Autodesk Fusion 360 part; units mm, degrees
note: some values were not read from the file. Set by a fixed rule: which sketch regions a step uses.
(part 2 of 3)
sketch "Schizzo100" plane through (0, 18, -31.1769) normal (0, 0.5, -0.866025) x (0, -0.866025, -0.5)
  circle A0 centre (14.956, -5.5311) radius 0.5023
  circle A1 centre (14.956, -9.1821) radius 0.5023
  circle A2 centre (14.956, -12.833) radius 0.5023
  circle A3 centre (14.956, -16.4839) radius 0.5023
  circle A4 centre (14.956, -20.1349) radius 0.5023
  circle A5 centre (14.956, -23.7858) radius 0.5023
  circle A6 centre (14.956, -27.4367) radius 0.5023
  circle A7 centre (14.956, -31.0877) radius 0.5023
  circle A8 centre (14.956, -34.7386) radius 0.5023
  circle A9 centre (14.956, -38.3895) radius 0.5023
  circle A10 centre (14.956, -42.0405) radius 0.5023
  circle A11 centre (14.956, -45.6914) radius 0.5023
  circle A12 centre (14.956, -49.3423) radius 0.5023
  circle A13 centre (14.956, -52.9933) radius 0.5023
  circle A14 centre (14.956, -56.6442) radius 0.5023
  circle A15 centre (14.956, -60.2951) radius 0.5023
  circle A16 centre (14.956, -63.9461) radius 0.5023
  circle A17 centre (14.956, -67.597) radius 0.5023
  circle A18 centre (14.956, -71.248) radius 0.5023
  circle A19 centre (14.956, -74.8989) radius 0.5023
  circle A20 centre (14.956, -78.5498) radius 0.5023
  circle A21 centre (14.956, -82.2008) radius 0.5023
  circle A22 centre (14.956, -85.8517) radius 0.5023
  circle A23 centre (14.956, -89.5026) radius 0.5023
  circle A24 centre (14.956, -93.1536) radius 0.5023
  circle A25 centre (14.956, -96.8045) radius 0.5023
  circle A26 centre (14.956, -100.4554) radius 0.5023
  circle A27 centre (14.956, -104.1064) radius 0.5023
  circle A28 centre (14.956, -107.7573) radius 0.5023
  circle A29 centre (14.956, -111.4082) radius 0.5023
  circle A30 centre (14.956, -115.0592) radius 0.5023
  circle A31 centre (14.956, -118.7101) radius 0.5023
  circle A32 centre (14.956, -122.361) radius 0.5023
  circle A33 centre (14.956, -126.012) radius 0.5023
  circle A34 centre (14.956, -129.6629) radius 0.5023
  circle A35 centre (14.956, -133.3138) radius 0.5023
  circle A36 centre (14.956, -136.9648) radius 0.5023
  circle A37 centre (14.956, -140.6157) radius 0.5023
  circle A38 centre (14.956, -144.2667) radius 0.5023
  circle A39 centre (14.956, -147.9176) radius 0.5023
  circle A40 centre (14.956, -151.5685) radius 0.5023
  circle A41 centre (14.956, -155.2195) radius 0.5023
  circle A42 centre (14.956, -158.8704) radius 0.5023
  circle A43 centre (14.956, -162.5213) radius 0.5023
  circle A44 centre (14.956, -166.1723) radius 0.5023
  circle A45 centre (14.956, -169.8232) radius 0.5023
  circle A46 centre (14.956, -173.4741) radius 0.5023
  circle A47 centre (14.956, -177.1251) radius 0.5023
  circle A48 centre (14.956, -180.776) radius 0.5023
  circle A49 centre (14.956, -184.4269) radius 0.5023
  circle A50 centre (14.956, -188.0779) radius 0.5023
  circle A51 centre (14.956, -191.7288) radius 0.5023
  circle A52 centre (14.956, -195.3797) radius 0.5023
  circle A53 centre (14.956, -199.0307) radius 0.5023
  circle A54 centre (14.956, -202.6816) radius 0.5023
  circle A55 centre (14.956, -206.3325) radius 0.5023
  circle A56 centre (14.956, -209.9835) radius 0.5023
  circle A57 centre (14.956, -213.6344) radius 0.5023
  circle A58 centre (14.956, -217.2853) radius 0.5023
  circle A59 centre (14.956, -220.9363) radius 0.5023
  circle A60 centre (14.956, -224.5872) radius 0.5023
  circle A61 centre (13.1468, -7.3404) radius 0.5023
  circle A62 centre (13.1468, -10.9913) radius 0.5023
  circle A63 centre (13.1468, -14.6422) radius 0.5023
  circle A64 centre (13.1468, -18.2932) radius 0.5023
  circle A65 centre (13.1468, -21.9441) radius 0.5023
  circle A66 centre (13.1468, -25.595) radius 0.5023
  circle A67 centre (13.1468, -29.246) radius 0.5023
  circle A68 centre (13.1468, -32.8969) radius 0.5023
  circle A69 centre (13.1468, -36.5478) radius 0.5023
  circle A70 centre (13.1468, -40.1988) radius 0.5023
  circle A71 centre (13.1468, -43.8497) radius 0.5023
  circle A72 centre (13.1468, -47.5006) radius 0.5023
  circle A73 centre (13.1468, -51.1516) radius 0.5023
  circle A74 centre (13.1468, -54.8025) radius 0.5023
  circle A75 centre (13.1468, -58.4534) radius 0.5023
  circle A76 centre (13.1468, -62.1044) radius 0.5023
  circle A77 centre (13.1468, -65.7553) radius 0.5023
  circle A78 centre (13.1468, -69.4062) radius 0.5023
  circle A79 centre (13.1468, -73.0572) radius 0.5023
  circle A80 centre (13.1468, -76.7081) radius 0.5023
  circle A81 centre (13.1468, -80.3591) radius 0.5023
  circle A82 centre (13.1468, -84.01) radius 0.5023
  circle A83 centre (13.1468, -87.6609) radius 0.5023
  circle A84 centre (13.1468, -91.3119) radius 0.5023
  circle A85 centre (13.1468, -94.9628) radius 0.5023
  circle A86 centre (13.1468, -98.6137) radius 0.5023
  circle A87 centre (13.1468, -102.2647) radius 0.5023
  circle A88 centre (13.1468, -105.9156) radius 0.5023
  circle A89 centre (13.1468, -109.5665) radius 0.5023
  circle A90 centre (13.1468, -113.2175) radius 0.5023
  circle A91 centre (13.1468, -116.8684) radius 0.5023
  circle A92 centre (13.1468, -120.5193) radius 0.5023
  circle A93 centre (13.1468, -124.1703) radius 0.5023
  circle A94 centre (13.1468, -127.8212) radius 0.5023
  circle A95 centre (13.1468, -131.4721) radius 0.5023
  circle A96 centre (13.1468, -135.1231) radius 0.5023
  circle A97 centre (13.1468, -138.774) radius 0.5023
  circle A98 centre (13.1468, -142.4249) radius 0.5023
  circle A99 centre (13.1468, -146.0759) radius 0.5023
  circle A100 centre (13.1468, -149.7268) radius 0.5023
  circle A101 centre (13.1468, -153.3778) radius 0.5023
  circle A102 centre (13.1468, -157.0287) radius 0.5023
  circle A103 centre (13.1468, -160.6796) radius 0.5023
  circle A104 centre (13.1468, -164.3306) radius 0.5023
  circle A105 centre (13.1468, -167.9815) radius 0.5023
  circle A106 centre (13.1468, -171.6324) radius 0.5023
  circle A107 centre (13.1468, -175.2834) radius 0.5023
  circle A108 centre (13.1468, -178.9343) radius 0.5023
  circle A109 centre (13.1468, -182.5852) radius 0.5023
  circle A110 centre (13.1468, -186.2362) radius 0.5023
  circle A111 centre (13.1468, -189.8871) radius 0.5023
  circle A112 centre (13.1468, -193.538) radius 0.5023
  circle A113 centre (13.1468, -197.189) radius 0.5023
  circle A114 centre (13.1468, -200.8399) radius 0.5023
  circle A115 centre (13.1468, -204.4908) radius 0.5023
  circle A116 centre (13.1468, -208.1418) radius 0.5023
  circle A117 centre (13.1468, -211.7927) radius 0.5023
  circle A118 centre (13.1468, -215.4436) radius 0.5023
  circle A119 centre (13.1468, -219.0946) radius 0.5023
  circle A120 centre (13.1468, -222.7455) radius 0.5023
  circle A121 centre (10.6739, -5.5311) radius 0.5023
  circle A122 centre (10.6739, -9.1821) radius 0.5023
  circle A123 centre (10.6739, -12.833) radius 0.5023
  circle A124 centre (10.6739, -16.4839) radius 0.5023
  circle A125 centre (10.6739, -20.1349) radius 0.5023
  circle A126 centre (10.6739, -23.7858) radius 0.5023
  circle A127 centre (10.6739, -27.4367) radius 0.5023
  circle A128 centre (10.6739, -31.0877) radius 0.5023
  circle A129 centre (10.6739, -34.7386) radius 0.5023
  circle A130 centre (10.6739, -38.3895) radius 0.5023
  circle A131 centre (10.6739, -42.0405) radius 0.5023
  circle A132 centre (10.6739, -45.6914) radius 0.5023
  circle A133 centre (10.6739, -49.3423) radius 0.5023
  circle A134 centre (10.6739, -52.9933) radius 0.5023
  circle A135 centre (10.6739, -56.6442) radius 0.5023
  circle A136 centre (10.6739, -60.2951) radius 0.5023
  circle A137 centre (10.6739, -63.9461) radius 0.5023
  circle A138 centre (10.6739, -67.597) radius 0.5023
  circle A139 centre (10.6739, -71.248) radius 0.5023
  circle A140 centre (10.6739, -74.8989) radius 0.5023
  circle A141 centre (10.6739, -78.5498) radius 0.5023
  circle A142 centre (10.6739, -82.2008) radius 0.5023
  circle A143 centre (10.6739, -85.8517) radius 0.5023
  circle A144 centre (10.6739, -89.5026) radius 0.5023
  circle A145 centre (10.6739, -93.1536) radius 0.5023
  circle A146 centre (10.6739, -96.8045) radius 0.5023
  circle A147 centre (10.6739, -100.4554) radius 0.5023
  circle A148 centre (10.6739, -104.1064) radius 0.5023
  circle A149 centre (10.6739, -107.7573) radius 0.5023
  circle A150 centre (10.6739, -111.4082) radius 0.5023
  circle A151 centre (10.6739, -115.0592) radius 0.5023
  circle A152 centre (10.6739, -118.7101) radius 0.5023
  circle A153 centre (10.6739, -122.361) radius 0.5023
  circle A154 centre (10.6739, -126.012) radius 0.5023
  circle A155 centre (10.6739, -129.6629) radius 0.5023
  circle A156 centre (10.6739, -133.3138) radius 0.5023
  circle A157 centre (10.6739, -136.9648) radius 0.5023
  circle A158 centre (10.6739, -140.6157) radius 0.5023
  circle A159 centre (10.6739, -144.2667) radius 0.5023
  circle A160 centre (10.6739, -147.9176) radius 0.5023
  circle A161 centre (10.6739, -151.5685) radius 0.5023
  circle A162 centre (10.6739, -155.2195) radius 0.5023
  circle A163 centre (10.6739, -158.8704) radius 0.5023
  circle A164 centre (10.6739, -162.5213) radius 0.5023
  circle A165 centre (10.6739, -166.1723) radius 0.5023
  circle A166 centre (10.6739, -169.8232) radius 0.5023
  circle A167 centre (10.6739, -173.4741) radius 0.5023
  circle A168 centre (10.6739, -177.1251) radius 0.5023
  circle A169 centre (10.6739, -180.776) radius 0.5023
  circle A170 centre (10.6739, -184.4269) radius 0.5023
  circle A171 centre (10.6739, -188.0779) radius 0.5023
  circle A172 centre (10.6739, -191.7288) radius 0.5023
  circle A173 centre (10.6739, -195.3797) radius 0.5023
  circle A174 centre (10.6739, -199.0307) radius 0.5023
  circle A175 centre (10.6739, -202.6816) radius 0.5023
  circle A176 centre (10.6739, -206.3325) radius 0.5023
  circle A177 centre (10.6739, -209.9835) radius 0.5023
  circle A178 centre (10.6739, -213.6344) radius 0.5023
  circle A179 centre (10.6739, -217.2853) radius 0.5023
  circle A180 centre (10.6739, -220.9363) radius 0.5023
  circle A181 centre (10.6739, -224.5872) radius 0.5023
  circle A182 centre (8.8647, -7.3404) radius 0.5023
  circle A183 centre (8.8647, -10.9913) radius 0.5023
  circle A184 centre (8.8647, -14.6422) radius 0.5023
  circle A185 centre (8.8647, -18.2932) radius 0.5023
  circle A186 centre (8.8647, -21.9441) radius 0.5023
  circle A187 centre (8.8647, -25.595) radius 0.5023
  circle A188 centre (8.8647, -29.246) radius 0.5023
  circle A189 centre (8.8647, -32.8969) radius 0.5023
  circle A190 centre (8.8647, -36.5478) radius 0.5023
  circle A191 centre (8.8647, -40.1988) radius 0.5023
  circle A192 centre (8.8647, -43.8497) radius 0.5023
  circle A193 centre (8.8647, -47.5006) radius 0.5023
  circle A194 centre (8.8647, -51.1516) radius 0.5023
  circle A195 centre (8.8647, -54.8025) radius 0.5023
  circle A196 centre (8.8647, -58.4534) radius 0.5023
  circle A197 centre (8.8647, -62.1044) radius 0.5023
  circle A198 centre (8.8647, -65.7553) radius 0.5023
  circle A199 centre (8.8647, -69.4062) radius 0.5023
  circle A200 centre (8.8647, -73.0572) radius 0.5023
  circle A201 centre (8.8647, -76.7081) radius 0.5023
  circle A202 centre (8.8647, -80.3591) radius 0.5023
  circle A203 centre (8.8647, -84.01) radius 0.5023
  circle A204 centre (8.8647, -87.6609) radius 0.5023
  circle A205 centre (8.8647, -91.3119) radius 0.5023
  circle A206 centre (8.8647, -94.9628) radius 0.5023
  circle A207 centre (8.8647, -98.6137) radius 0.5023
  circle A208 centre (8.8647, -102.2647) radius 0.5023
  circle A209 centre (8.8647, -105.9156) radius 0.5023
  circle A210 centre (8.8647, -109.5665) radius 0.5023
  circle A211 centre (8.8647, -113.2175) radius 0.5023
  circle A212 centre (8.8647, -116.8684) radius 0.5023
  circle A213 centre (8.8647, -120.5193) radius 0.5023
  circle A214 centre (8.8647, -124.1703) radius 0.5023
  circle A215 centre (8.8647, -127.8212) radius 0.5023
  circle A216 centre (8.8647, -131.4721) radius 0.5023
  circle A217 centre (8.8647, -135.1231) radius 0.5023
  circle A218 centre (8.8647, -138.774) radius 0.5023
  circle A219 centre (8.8647, -142.4249) radius 0.5023
  circle A220 centre (8.8647, -146.0759) radius 0.5023
  circle A221 centre (8.8647, -149.7268) radius 0.5023
  circle A222 centre (8.8647, -153.3778) radius 0.5023
  circle A223 centre (8.8647, -157.0287) radius 0.5023
  circle A224 centre (8.8647, -160.6796) radius 0.5023
  circle A225 centre (8.8647, -164.3306) radius 0.5023
  circle A226 centre (8.8647, -167.9815) radius 0.5023
  circle A227 centre (8.8647, -171.6324) radius 0.5023
  circle A228 centre (8.8647, -175.2834) radius 0.5023
  circle A229 centre (8.8647, -178.9343) radius 0.5023
  circle A230 centre (8.8647, -182.5852) radius 0.5023
  circle A231 centre (8.8647, -186.2362) radius 0.5023
  circle A232 centre (8.8647, -189.8871) radius 0.5023
  circle A233 centre (8.8647, -193.538) radius 0.5023
  circle A234 centre (8.8647, -197.189) radius 0.5023
  circle A235 centre (8.8647, -200.8399) radius 0.5023
  circle A236 centre (8.8647, -204.4908) radius 0.5023
  circle A237 centre (8.8647, -208.1418) radius 0.5023
  circle A238 centre (8.8647, -211.7927) radius 0.5023
  circle A239 centre (8.8647, -215.4436) radius 0.5023
  circle A240 centre (8.8647, -219.0946) radius 0.5023
  circle A241 centre (8.8647, -222.7455) radius 0.5023
  circle A242 centre (6.3918, -5.5311) radius 0.5023
  circle A243 centre (6.3918, -9.1821) radius 0.5023
  circle A244 centre (6.3918, -12.833) radius 0.5023
  circle A245 centre (6.3918, -16.4839) radius 0.5023
  circle A246 centre (6.3918, -20.1349) radius 0.5023
  circle A247 centre (6.3918, -23.7858) radius 0.5023
  circle A248 centre (6.3918, -27.4367) radius 0.5023
  circle A249 centre (6.3918, -31.0877) radius 0.5023
  circle A250 centre (6.3918, -34.7386) radius 0.5023
  circle A251 centre (6.3918, -38.3895) radius 0.5023
  circle A252 centre (6.3918, -42.0405) radius 0.5023
  circle A253 centre (6.3918, -45.6914) radius 0.5023
  circle A254 centre (6.3918, -49.3423) radius 0.5023
  circle A255 centre (6.3918, -52.9933) radius 0.5023
  circle A256 centre (6.3918, -56.6442) radius 0.5023
  circle A257 centre (6.3918, -60.2951) radius 0.5023
  circle A258 centre (6.3918, -63.9461) radius 0.5023
  circle A259 centre (6.3918, -67.597) radius 0.5023
  circle A260 centre (6.3918, -71.248) radius 0.5023
  circle A261 centre (6.3918, -74.8989) radius 0.5023
  circle A262 centre (6.3918, -78.5498) radius 0.5023
  circle A263 centre (6.3918, -82.2008) radius 0.5023
  circle A264 centre (6.3918, -85.8517) radius 0.5023
  circle A265 centre (6.3918, -89.5026) radius 0.5023
  circle A266 centre (6.3918, -93.1536) radius 0.5023
  circle A267 centre (6.3918, -96.8045) radius 0.5023
  circle A268 centre (6.3918, -100.4554) radius 0.5023
  circle A269 centre (6.3918, -104.1064) radius 0.5023
  circle A270 centre (6.3918, -107.7573) radius 0.5023
  circle A271 centre (6.3918, -111.4082) radius 0.5023
  circle A272 centre (6.3918, -115.0592) radius 0.5023
  circle A273 centre (6.3918, -118.7101) radius 0.5023
  circle A274 centre (6.3918, -122.361) radius 0.5023
  circle A275 centre (6.3918, -126.012) radius 0.5023
  circle A276 centre (6.3918, -129.6629) radius 0.5023
  circle A277 centre (6.3918, -133.3138) radius 0.5023
  circle A278 centre (6.3918, -136.9648) radius 0.5023
  circle A279 centre (6.3918, -140.6157) radius 0.5023
  circle A280 centre (6.3918, -144.2667) radius 0.5023
  circle A281 centre (6.3918, -147.9176) radius 0.5023
  circle A282 centre (6.3918, -151.5685) radius 0.5023
  circle A283 centre (6.3918, -155.2195) radius 0.5023
  circle A284 centre (6.3918, -158.8704) radius 0.5023
  circle A285 centre (6.3918, -162.5213) radius 0.5023
  circle A286 centre (6.3918, -166.1723) radius 0.5023
  circle A287 centre (6.3918, -169.8232) radius 0.5023
  circle A288 centre (6.3918, -173.4741) radius 0.5023
  circle A289 centre (6.3918, -177.1251) radius 0.5023
  circle A290 centre (6.3918, -180.776) radius 0.5023
  circle A291 centre (6.3918, -184.4269) radius 0.5023
  circle A292 centre (6.3918, -188.0779) radius 0.5023
  circle A293 centre (6.3918, -191.7288) radius 0.5023
  circle A294 centre (6.3918, -195.3797) radius 0.5023
  circle A295 centre (6.3918, -199.0307) radius 0.5023
  circle A296 centre (6.3918, -202.6816) radius 0.5023
  circle A297 centre (6.3918, -206.3325) radius 0.5023
  circle A298 centre (6.3918, -209.9835) radius 0.5023
  circle A299 centre (6.3918, -213.6344) radius 0.5023
  circle A300 centre (6.3918, -217.2853) radius 0.5023
  circle A301 centre (6.3918, -220.9363) radius 0.5023
  circle A302 centre (6.3918, -224.5872) radius 0.5023
  circle A303 centre (4.5826, -7.3404) radius 0.5023
  circle A304 centre (4.5826, -10.9913) radius 0.5023
  circle A305 centre (4.5826, -14.6422) radius 0.5023
  circle A306 centre (4.5826, -18.2932) radius 0.5023
  circle A307 centre (4.5826, -21.9441) radius 0.5023
  circle A308 centre (4.5826, -25.595) radius 0.5023
  circle A309 centre (4.5826, -29.246) radius 0.5023
  circle A310 centre (4.5826, -32.8969) radius 0.5023
  circle A311 centre (4.5826, -36.5478) radius 0.5023
  circle A312 centre (4.5826, -40.1988) radius 0.5023
  circle A313 centre (4.5826, -43.8497) radius 0.5023
  circle A314 centre (4.5826, -47.5006) radius 0.5023
  circle A315 centre (4.5826, -51.1516) radius 0.5023
  circle A316 centre (4.5826, -54.8025) radius 0.5023
  circle A317 centre (4.5826, -58.4534) radius 0.5023
  circle A318 centre (4.5826, -62.1044) radius 0.5023
  circle A319 centre (4.5826, -65.7553) radius 0.5023
  circle A320 centre (4.5826, -69.4062) radius 0.5023
  circle A321 centre (4.5826, -73.0572) radius 0.5023
  circle A322 centre (4.5826, -76.7081) radius 0.5023
  circle A323 centre (4.5826, -80.3591) radius 0.5023
  circle A324 centre (4.5826, -84.01) radius 0.5023
  circle A325 centre (4.5826, -87.6609) radius 0.5023
  circle A326 centre (4.5826, -91.3119) radius 0.5023
  circle A327 centre (4.5826, -94.9628) radius 0.5023
  circle A328 centre (4.5826, -98.6137) radius 0.5023
  circle A329 centre (4.5826, -102.2647) radius 0.5023
  circle A330 centre (4.5826, -105.9156) radius 0.5023
  circle A331 centre (4.5826, -109.5665) radius 0.5023
  circle A332 centre (4.5826, -113.2175) radius 0.5023
  circle A333 centre (4.5826, -116.8684) radius 0.5023
  circle A334 centre (4.5826, -120.5193) radius 0.5023
  circle A335 centre (4.5826, -124.1703) radius 0.5023
  circle A336 centre (4.5826, -127.8212) radius 0.5023
  circle A337 centre (4.5826, -131.4721) radius 0.5023
  circle A338 centre (4.5826, -135.1231) radius 0.5023
  circle A339 centre (4.5826, -138.774) radius 0.5023
  circle A340 centre (4.5826, -142.4249) radius 0.5023
  circle A341 centre (4.5826, -146.0759) radius 0.5023
  circle A342 centre (4.5826, -149.7268) radius 0.5023
  circle A343 centre (4.5826, -153.3778) radius 0.5023
  circle A344 centre (4.5826, -157.0287) radius 0.5023
  circle A345 centre (4.5826, -160.6796) radius 0.5023
  circle A346 centre (4.5826, -164.3306) radius 0.5023
  circle A347 centre (4.5826, -167.9815) radius 0.5023
  circle A348 centre (4.5826, -171.6324) radius 0.5023
  circle A349 centre (4.5826, -175.2834) radius 0.5023
  circle A350 centre (4.5826, -178.9343) radius 0.5023
  circle A351 centre (4.5826, -182.5852) radius 0.5023
  circle A352 centre (4.5826, -186.2362) radius 0.5023
  circle A353 centre (4.5826, -189.8871) radius 0.5023
  circle A354 centre (4.5826, -193.538) radius 0.5023
  circle A355 centre (4.5826, -197.189) radius 0.5023
  circle A356 centre (4.5826, -200.8399) radius 0.5023
  circle A357 centre (4.5826, -204.4908) radius 0.5023
  circle A358 centre (4.5826, -208.1418) radius 0.5023
  circle A359 centre (4.5826, -211.7927) radius 0.5023
  circle A360 centre (4.5826, -215.4436) radius 0.5023
  circle A361 centre (4.5826, -219.0946) radius 0.5023
  circle A362 centre (4.5826, -222.7455) radius 0.5023
  circle A363 centre (2.1097, -5.5311) radius 0.5023
  circle A364 centre (2.1097, -9.1821) radius 0.5023
  circle A365 centre (2.1097, -12.833) radius 0.5023
  circle A366 centre (2.1097, -16.4839) radius 0.5023
  circle A367 centre (2.1097, -20.1349) radius 0.5023
  circle A368 centre (2.1097, -23.7858) radius 0.5023
  circle A369 centre (2.1097, -27.4367) radius 0.5023
  circle A370 centre (2.1097, -31.0877) radius 0.5023
  circle A371 centre (2.1097, -34.7386) radius 0.5023
  circle A372 centre (2.1097, -38.3895) radius 0.5023
  circle A373 centre (2.1097, -42.0405) radius 0.5023
  circle A374 centre (2.1097, -45.6914) radius 0.5023
  circle A375 centre (2.1097, -49.3423) radius 0.5023
  circle A376 centre (2.1097, -52.9933) radius 0.5023
  circle A377 centre (2.1097, -56.6442) radius 0.5023
  circle A378 centre (2.1097, -60.2951) radius 0.5023
  circle A379 centre (2.1097, -63.9461) radius 0.5023
  circle A380 centre (2.1097, -67.597) radius 0.5023
  circle A381 centre (2.1097, -71.248) radius 0.5023
  circle A382 centre (2.1097, -74.8989) radius 0.5023
  circle A383 centre (2.1097, -78.5498) radius 0.5023
  circle A384 centre (2.1097, -82.2008) radius 0.5023
  circle A385 centre (2.1097, -85.8517) radius 0.5023
  circle A386 centre (2.1097, -89.5026) radius 0.5023
  circle A387 centre (2.1097, -93.1536) radius 0.5023
  circle A388 centre (2.1097, -96.8045) radius 0.5023
  circle A389 centre (2.1097, -100.4554) radius 0.5023
  circle A390 centre (2.1097, -104.1064) radius 0.5023
  circle A391 centre (2.1097, -107.7573) radius 0.5023
  circle A392 centre (2.1097, -111.4082) radius 0.5023
  circle A393 centre (2.1097, -115.0592) radius 0.5023
  circle A394 centre (2.1097, -118.7101) radius 0.5023
  circle A395 centre (2.1097, -122.361) radius 0.5023
  circle A396 centre (2.1097, -126.012) radius 0.5023
  circle A397 centre (2.1097, -129.6629) radius 0.5023
  circle A398 centre (2.1097, -133.3138) radius 0.5023
  circle A399 centre (2.1097, -136.9648) radius 0.5023
  circle A400 centre (2.1097, -140.6157) radius 0.5023
  circle A401 centre (2.1097, -144.2667) radius 0.5023
  circle A402 centre (2.1097, -147.9176) radius 0.5023
  circle A403 centre (2.1097, -151.5685) radius 0.5023
  circle A404 centre (2.1097, -155.2195) radius 0.5023
  circle A405 centre (2.1097, -158.8704) radius 0.5023
  circle A406 centre (2.1097, -162.5213) radius 0.5023
  circle A407 centre (2.1097, -166.1723) radius 0.5023
  circle A408 centre (2.1097, -169.8232) radius 0.5023
  circle A409 centre (2.1097, -173.4741) radius 0.5023
  circle A410 centre (2.1097, -177.1251) radius 0.5023
  circle A411 centre (2.1097, -180.776) radius 0.5023
  circle A412 centre (2.1097, -184.4269) radius 0.5023
  circle A413 centre (2.1097, -188.0779) radius 0.5023
  circle A414 centre (2.1097, -191.7288) radius 0.5023
  circle A415 centre (2.1097, -195.3797) radius 0.5023
  circle A416 centre (2.1097, -199.0307) radius 0.5023
  circle A417 centre (2.1097, -202.6816) radius 0.5023
  circle A418 centre (2.1097, -206.3325) radius 0.5023
  circle A419 centre (2.1097, -209.9835) radius 0.5023
  circle A420 centre (2.1097, -213.6344) radius 0.5023
  circle A421 centre (2.1097, -217.2853) radius 0.5023
  circle A422 centre (2.1097, -220.9363) radius 0.5023
  circle A423 centre (2.1097, -224.5872) radius 0.5023
  circle A424 centre (0.3005, -7.3404) radius 0.5023
  circle A425 centre (0.3005, -10.9913) radius 0.5023
  circle A426 centre (0.3005, -14.6422) radius 0.5023
  circle A427 centre (0.3005, -18.2932) radius 0.5023
  circle A428 centre (0.3005, -21.9441) radius 0.5023
  circle A429 centre (0.3005, -25.595) radius 0.5023
  circle A430 centre (0.3005, -29.246) radius 0.5023
  circle A431 centre (0.3005, -32.8969) radius 0.5023
  circle A432 centre (0.3005, -36.5478) radius 0.5023
  circle A433 centre (0.3005, -40.1988) radius 0.5023
  circle A434 centre (0.3005, -43.8497) radius 0.5023
  circle A435 centre (0.3005, -47.5006) radius 0.5023
  circle A436 centre (0.3005, -51.1516) radius 0.5023
  circle A437 centre (0.3005, -54.8025) radius 0.5023
  circle A438 centre (0.3005, -58.4534) radius 0.5023
  circle A439 centre (0.3005, -62.1044) radius 0.5023
  circle A440 centre (0.3005, -65.7553) radius 0.5023
  circle A441 centre (0.3005, -69.4062) radius 0.5023
  circle A442 centre (0.3005, -73.0572) radius 0.5023
  circle A443 centre (0.3005, -76.7081) radius 0.5023
  circle A444 centre (0.3005, -80.3591) radius 0.5023
  circle A445 centre (0.3005, -84.01) radius 0.5023
  circle A446 centre (0.3005, -87.6609) radius 0.5023
  circle A447 centre (0.3005, -91.3119) radius 0.5023
  circle A448 centre (0.3005, -94.9628) radius 0.5023
  circle A449 centre (0.3005, -98.6137) radius 0.5023
  circle A450 centre (0.3005, -102.2647) radius 0.5023
  circle A451 centre (0.3005, -105.9156) radius 0.5023
  circle A452 centre (0.3005, -109.5665) radius 0.5023
  circle A453 centre (0.3005, -113.2175) radius 0.5023
  circle A454 centre (0.3005, -116.8684) radius 0.5023
  circle A455 centre (0.3005, -120.5193) radius 0.5023
  circle A456 centre (0.3005, -124.1703) radius 0.5023
  circle A457 centre (0.3005, -127.8212) radius 0.5023
  circle A458 centre (0.3005, -131.4721) radius 0.5023
  circle A459 centre (0.3005, -135.1231) radius 0.5023
  circle A460 centre (0.3005, -138.774) radius 0.5023
  circle A461 centre (0.3005, -142.4249) radius 0.5023
  circle A462 centre (0.3005, -146.0759) radius 0.5023
  circle A463 centre (0.3005, -149.7268) radius 0.5023
  circle A464 centre (0.3005, -153.3778) radius 0.5023
  circle A465 centre (0.3005, -157.0287) radius 0.5023
  circle A466 centre (0.3005, -160.6796) radius 0.5023
  circle A467 centre (0.3005, -164.3306) radius 0.5023
  circle A468 centre (0.3005, -167.9815) radius 0.5023
  circle A469 centre (0.3005, -171.6324) radius 0.5023
  circle A470 centre (0.3005, -175.2834) radius 0.5023
  circle A471 centre (0.3005, -178.9343) radius 0.5023
  circle A472 centre (0.3005, -182.5852) radius 0.5023
  circle A473 centre (0.3005, -186.2362) radius 0.5023
  circle A474 centre (0.3005, -189.8871) radius 0.5023
  circle A475 centre (0.3005, -193.538) radius 0.5023
  circle A476 centre (0.3005, -197.189) radius 0.5023
  circle A477 centre (0.3005, -200.8399) radius 0.5023
  circle A478 centre (0.3005, -204.4908) radius 0.5023
  circle A479 centre (0.3005, -208.1418) radius 0.5023
  circle A480 centre (0.3005, -211.7927) radius 0.5023
  circle A481 centre (0.3005, -215.4436) radius 0.5023
  circle A482 centre (0.3005, -219.0946) radius 0.5023
  circle A483 centre (0.3005, -222.7455) radius 0.5023
  circle A484 centre (-2.1724, -5.5311) radius 0.5023
  circle A485 centre (-2.1724, -9.1821) radius 0.5023
  circle A486 centre (-2.1724, -12.833) radius 0.5023
  circle A487 centre (-2.1724, -16.4839) radius 0.5023
  circle A488 centre (-2.1724, -20.1349) radius 0.5023
  circle A489 centre (-2.1724, -23.7858) radius 0.5023
  circle A490 centre (-2.1724, -27.4367) radius 0.5023
  circle A491 centre (-2.1724, -31.0877) radius 0.5023
  circle A492 centre (-2.1724, -34.7386) radius 0.5023
  circle A493 centre (-2.1724, -38.3895) radius 0.5023
  circle A494 centre (-2.1724, -42.0405) radius 0.5023
  circle A495 centre (-2.1724, -45.6914) radius 0.5023
  circle A496 centre (-2.1724, -49.3423) radius 0.5023
  circle A497 centre (-2.1724, -52.9933) radius 0.5023
  circle A498 centre (-2.1724, -56.6442) radius 0.5023
  circle A499 centre (-2.1724, -60.2951) radius 0.5023
  circle A500 centre (-2.1724, -63.9461) radius 0.5023
  circle A501 centre (-2.1724, -67.597) radius 0.5023
  circle A502 centre (-2.1724, -71.248) radius 0.5023
  circle A503 centre (-2.1724, -74.8989) radius 0.5023
  circle A504 centre (-2.1724, -78.5498) radius 0.5023
  circle A505 centre (-2.1724, -82.2008) radius 0.5023
  circle A506 centre (-2.1724, -85.8517) radius 0.5023
  circle A507 centre (-2.1724, -89.5026) radius 0.5023
  circle A508 centre (-2.1724, -93.1536) radius 0.5023
  circle A509 centre (-2.1724, -96.8045) radius 0.5023
  circle A510 centre (-2.1724, -100.4554) radius 0.5023
  circle A511 centre (-2.1724, -104.1064) radius 0.5023
  circle A512 centre (-2.1724, -107.7573) radius 0.5023
  circle A513 centre (-2.1724, -111.4082) radius 0.5023
  circle A514 centre (-2.1724, -115.0592) radius 0.5023
  circle A515 centre (-2.1724, -118.7101) radius 0.5023
  circle A516 centre (-2.1724, -122.361) radius 0.5023
  circle A517 centre (-2.1724, -126.012) radius 0.5023
  circle A518 centre (-2.1724, -129.6629) radius 0.5023
  circle A519 centre (-2.1724, -133.3138) radius 0.5023
  circle A520 centre (-2.1724, -136.9648) radius 0.5023
  circle A521 centre (-2.1724, -140.6157) radius 0.5023
  circle A522 centre (-2.1724, -144.2667) radius 0.5023
  circle A523 centre (-2.1724, -147.9176) radius 0.5023
  circle A524 centre (-2.1724, -151.5685) radius 0.5023
  circle A525 centre (-2.1724, -155.2195) radius 0.5023
  circle A526 centre (-2.1724, -158.8704) radius 0.5023
  circle A527 centre (-2.1724, -162.5213) radius 0.5023
  circle A528 centre (-2.1724, -166.1723) radius 0.5023
  circle A529 centre (-2.1724, -169.8232) radius 0.5023
  circle A530 centre (-2.1724, -173.4741) radius 0.5023
  circle A531 centre (-2.1724, -177.1251) radius 0.5023
  circle A532 centre (-2.1724, -180.776) radius 0.5023
  circle A533 centre (-2.1724, -184.4269) radius 0.5023
  circle A534 centre (-2.1724, -188.0779) radius 0.5023
  circle A535 centre (-2.1724, -191.7288) radius 0.5023
  circle A536 centre (-2.1724, -195.3797) radius 0.5023
  circle A537 centre (-2.1724, -199.0307) radius 0.5023
  circle A538 centre (-2.1724, -202.6816) radius 0.5023
  circle A539 centre (-2.1724, -206.3325) radius 0.5023
  circle A540 centre (-2.1724, -209.9835) radius 0.5023
  circle A541 centre (-2.1724, -213.6344) radius 0.5023
  circle A542 centre (-2.1724, -217.2853) radius 0.5023
  circle A543 centre (-2.1724, -220.9363) radius 0.5023
  circle A544 centre (-2.1724, -224.5872) radius 0.5023
  circle A545 centre (-3.9816, -7.3404) radius 0.5023
  circle A546 centre (-3.9816, -10.9913) radius 0.5023
  circle A547 centre (-3.9816, -14.6422) radius 0.5023
  circle A548 centre (-3.9816, -18.2932) radius 0.5023
  circle A549 centre (-3.9816, -21.9441) radius 0.5023
  circle A550 centre (-3.9816, -25.595) radius 0.5023
  circle A551 centre (-3.9816, -29.246) radius 0.5023
  circle A552 centre (-3.9816, -32.8969) radius 0.5023
  circle A553 centre (-3.9816, -36.5478) radius 0.5023
  circle A554 centre (-3.9816, -40.1988) radius 0.5023
  circle A555 centre (-3.9816, -43.8497) radius 0.5023
  circle A556 centre (-3.9816, -47.5006) radius 0.5023
  circle A557 centre (-3.9816, -51.1516) radius 0.5023
  circle A558 centre (-3.9816, -54.8025) radius 0.5023
  circle A559 centre (-3.9816, -58.4534) radius 0.5023
  circle A560 centre (-3.9816, -62.1044) radius 0.5023
  circle A561 centre (-3.9816, -65.7553) radius 0.5023
  circle A562 centre (-3.9816, -69.4062) radius 0.5023
  circle A563 centre (-3.9816, -73.0572) radius 0.5023
  circle A564 centre (-3.9816, -76.7081) radius 0.5023
  circle A565 centre (-3.9816, -80.3591) radius 0.5023
  circle A566 centre (-3.9816, -84.01) radius 0.5023
  circle A567 centre (-3.9816, -87.6609) radius 0.5023
  circle A568 centre (-3.9816, -91.3119) radius 0.5023
  circle A569 centre (-3.9816, -94.9628) radius 0.5023
  circle A570 centre (-3.9816, -98.6137) radius 0.5023
  circle A571 centre (-3.9816, -102.2647) radius 0.5023
  circle A572 centre (-3.9816, -105.9156) radius 0.5023
  circle A573 centre (-3.9816, -109.5665) radius 0.5023
  circle A574 centre (-3.9816, -113.2175) radius 0.5023
  circle A575 centre (-3.9816, -116.8684) radius 0.5023
  circle A576 centre (-3.9816, -120.5193) radius 0.5023
  circle A577 centre (-3.9816, -124.1703) radius 0.5023
  circle A578 centre (-3.9816, -127.8212) radius 0.5023
  circle A579 centre (-3.9816, -131.4721) radius 0.5023
  circle A580 centre (-3.9816, -135.1231) radius 0.5023
  circle A581 centre (-3.9816, -138.774) radius 0.5023
  circle A582 centre (-3.9816, -142.4249) radius 0.5023
  circle A583 centre (-3.9816, -146.0759) radius 0.5023
  circle A584 centre (-3.9816, -149.7268) radius 0.5023
  circle A585 centre (-3.9816, -153.3778) radius 0.5023
  circle A586 centre (-3.9816, -157.0287) radius 0.5023
  circle A587 centre (-3.9816, -160.6796) radius 0.5023
  circle A588 centre (-3.9816, -164.3306) radius 0.5023
  circle A589 centre (-3.9816, -167.9815) radius 0.5023
  circle A590 centre (-3.9816, -171.6324) radius 0.5023
  circle A591 centre (-3.9816, -175.2834) radius 0.5023
  circle A592 centre (-3.9816, -178.9343) radius 0.5023
  circle A593 centre (-3.9816, -182.5852) radius 0.5023
  circle A594 centre (-3.9816, -186.2362) radius 0.5023
  circle A595 centre (-3.9816, -189.8871) radius 0.5023
  circle A596 centre (-3.9816, -193.538) radius 0.5023
  circle A597 centre (-3.9816, -197.189) radius 0.5023
  circle A598 centre (-3.9816, -200.8399) radius 0.5023
  circle A599 centre (-3.9816, -204.4908) radius 0.5023
  circle A600 centre (-3.9816, -208.1418) radius 0.5023
  circle A601 centre (-3.9816, -211.7927) radius 0.5023
  circle A602 centre (-3.9816, -215.4436) radius 0.5023
  circle A603 centre (-3.9816, -219.0946) radius 0.5023
  circle A604 centre (-3.9816, -222.7455) radius 0.5023
  circle A605 centre (-6.4544, -5.5311) radius 0.5023
  circle A606 centre (-6.4544, -9.1821) radius 0.5023
  circle A607 centre (-6.4544, -12.833) radius 0.5023
  circle A608 centre (-6.4544, -16.4839) radius 0.5023
  circle A609 centre (-6.4544, -20.1349) radius 0.5023
  circle A610 centre (-6.4544, -23.7858) radius 0.5023
  circle A611 centre (-6.4544, -27.4367) radius 0.5023
  circle A612 centre (-6.4544, -31.0877) radius 0.5023
  circle A613 centre (-6.4544, -34.7386) radius 0.5023
  circle A614 centre (-6.4544, -38.3895) radius 0.5023
  circle A615 centre (-6.4544, -42.0405) radius 0.5023
  circle A616 centre (-6.4544, -45.6914) radius 0.5023
  circle A617 centre (-6.4544, -49.3423) radius 0.5023
  circle A618 centre (-6.4544, -52.9933) radius 0.5023
  circle A619 centre (-6.4544, -56.6442) radius 0.5023
  circle A620 centre (-6.4544, -60.2951) radius 0.5023
  circle A621 centre (-6.4544, -63.9461) radius 0.5023
  circle A622 centre (-6.4544, -67.597) radius 0.5023
  circle A623 centre (-6.4544, -71.248) radius 0.5023
  circle A624 centre (-6.4544, -74.8989) radius 0.5023
  circle A625 centre (-6.4544, -78.5498) radius 0.5023
  circle A626 centre (-6.4544, -82.2008) radius 0.5023
  circle A627 centre (-6.4544, -85.8517) radius 0.5023
  circle A628 centre (-6.4544, -89.5026) radius 0.5023
  circle A629 centre (-6.4544, -93.1536) radius 0.5023
  circle A630 centre (-6.4544, -96.8045) radius 0.5023
  circle A631 centre (-6.4544, -100.4554) radius 0.5023
  circle A632 centre (-6.4544, -104.1064) radius 0.5023
  circle A633 centre (-6.4544, -107.7573) radius 0.5023
  circle A634 centre (-6.4544, -111.4082) radius 0.5023
  circle A635 centre (-6.4544, -115.0592) radius 0.5023
  circle A636 centre (-6.4544, -118.7101) radius 0.5023
  circle A637 centre (-6.4544, -122.361) radius 0.5023
  circle A638 centre (-6.4544, -126.012) radius 0.5023
  circle A639 centre (-6.4544, -129.6629) radius 0.5023
  circle A640 centre (-6.4544, -133.3138) radius 0.5023
  circle A641 centre (-6.4544, -136.9648) radius 0.5023
  circle A642 centre (-6.4544, -140.6157) radius 0.5023
  circle A643 centre (-6.4544, -144.2667) radius 0.5023
  circle A644 centre (-6.4544, -147.9176) radius 0.5023
  circle A645 centre (-6.4544, -151.5685) radius 0.5023
  circle A646 centre (-6.4544, -155.2195) radius 0.5023
  circle A647 centre (-6.4544, -158.8704) radius 0.5023
  circle A648 centre (-6.4544, -162.5213) radius 0.5023
  circle A649 centre (-6.4544, -166.1723) radius 0.5023
  circle A650 centre (-6.4544, -169.8232) radius 0.5023
  circle A651 centre (-6.4544, -173.4741) radius 0.5023
  circle A652 centre (-6.4544, -177.1251) radius 0.5023
  circle A653 centre (-6.4544, -180.776) radius 0.5023
  circle A654 centre (-6.4544, -184.4269) radius 0.5023
  circle A655 centre (-6.4544, -188.0779) radius 0.5023
  circle A656 centre (-6.4544, -191.7288) radius 0.5023
  circle A657 centre (-6.4544, -195.3797) radius 0.5023
  circle A658 centre (-6.4544, -199.0307) radius 0.5023
  circle A659 centre (-6.4544, -202.6816) radius 0.5023
  circle A660 centre (-6.4544, -206.3325) radius 0.5023
  circle A661 centre (-6.4544, -209.9835) radius 0.5023
  circle A662 centre (-6.4544, -213.6344) radius 0.5023
  circle A663 centre (-6.4544, -217.2853) radius 0.5023
  circle A664 centre (-6.4544, -220.9363) radius 0.5023
  circle A665 centre (-6.4544, -224.5872) radius 0.5023
  circle A666 centre (-8.2637, -7.3404) radius 0.5023
  circle A667 centre (-8.2637, -10.9913) radius 0.5023
  circle A668 centre (-8.2637, -14.6422) radius 0.5023
  circle A669 centre (-8.2637, -18.2932) radius 0.5023
  circle A670 centre (-8.2637, -21.9441) radius 0.5023
  circle A671 centre (-8.2637, -25.595) radius 0.5023
  circle A672 centre (-8.2637, -29.246) radius 0.5023
  circle A673 centre (-8.2637, -32.8969) radius 0.5023
  circle A674 centre (-8.2637, -36.5478) radius 0.5023
  circle A675 centre (-8.2637, -40.1988) radius 0.5023
  circle A676 centre (-8.2637, -43.8497) radius 0.5023
  circle A677 centre (-8.2637, -47.5006) radius 0.5023
  circle A678 centre (-8.2637, -51.1516) radius 0.5023
  circle A679 centre (-8.2637, -54.8025) radius 0.5023
  circle A680 centre (-8.2637, -58.4534) radius 0.5023
  circle A681 centre (-8.2637, -62.1044) radius 0.5023
  circle A682 centre (-8.2637, -65.7553) radius 0.5023
  circle A683 centre (-8.2637, -69.4062) radius 0.5023
  circle A684 centre (-8.2637, -73.0572) radius 0.5023
  circle A685 centre (-8.2637, -76.7081) radius 0.5023
  circle A686 centre (-8.2637, -80.3591) radius 0.5023
  circle A687 centre (-8.2637, -84.01) radius 0.5023
  circle A688 centre (-8.2637, -87.6609) radius 0.5023
  circle A689 centre (-8.2637, -91.3119) radius 0.5023
  circle A690 centre (-8.2637, -94.9628) radius 0.5023
  circle A691 centre (-8.2637, -98.6137) radius 0.5023
  circle A692 centre (-8.2637, -102.2647) radius 0.5023
  circle A693 centre (-8.2637, -105.9156) radius 0.5023
  circle A694 centre (-8.2637, -109.5665) radius 0.5023
  circle A695 centre (-8.2637, -113.2175) radius 0.5023
  circle A696 centre (-8.2637, -116.8684) radius 0.5023
  circle A697 centre (-8.2637, -120.5193) radius 0.5023
  circle A698 centre (-8.2637, -124.1703) radius 0.5023
  circle A699 centre (-8.2637, -127.8212) radius 0.5023
  circle A700 centre (-8.2637, -131.4721) radius 0.5023
  circle A701 centre (-8.2637, -135.1231) radius 0.5023
  circle A702 centre (-8.2637, -138.774) radius 0.5023
  circle A703 centre (-8.2637, -142.4249) radius 0.5023
  circle A704 centre (-8.2637, -146.0759) radius 0.5023
  circle A705 centre (-8.2637, -149.7268) radius 0.5023
  circle A706 centre (-8.2637, -153.3778) radius 0.5023
  circle A707 centre (-8.2637, -157.0287) radius 0.5023
  circle A708 centre (-8.2637, -160.6796) radius 0.5023
  circle A709 centre (-8.2637, -164.3306) radius 0.5023
  circle A710 centre (-8.2637, -167.9815) radius 0.5023
  circle A711 centre (-8.2637, -171.6324) radius 0.5023
  circle A712 centre (-8.2637, -175.2834) radius 0.5023
  circle A713 centre (-8.2637, -178.9343) radius 0.5023
  circle A714 centre (-8.2637, -182.5852) radius 0.5023
  circle A715 centre (-8.2637, -186.2362) radius 0.5023
  circle A716 centre (-8.2637, -189.8871) radius 0.5023
  circle A717 centre (-8.2637, -193.538) radius 0.5023
  circle A718 centre (-8.2637, -197.189) radius 0.5023
  circle A719 centre (-8.2637, -200.8399) radius 0.5023
  circle A720 centre (-8.2637, -204.4908) radius 0.5023
  circle A721 centre (-8.2637, -208.1418) radius 0.5023
  circle A722 centre (-8.2637, -211.7927) radius 0.5023
  circle A723 centre (-8.2637, -215.4436) radius 0.5023
  circle A724 centre (-8.2637, -219.0946) radius 0.5023
  circle A725 centre (-8.2637, -222.7455) radius 0.5023
  circle A726 centre (-10.7365, -5.5311) radius 0.5023
  circle A727 centre (-10.7365, -9.1821) radius 0.5023
  circle A728 centre (-10.7365, -12.833) radius 0.5023
  circle A729 centre (-10.7365, -16.4839) radius 0.5023
  circle A730 centre (-10.7365, -20.1349) radius 0.5023
  circle A731 centre (-10.7365, -23.7858) radius 0.5023
  circle A732 centre (-10.7365, -27.4367) radius 0.5023
  circle A733 centre (-10.7365, -31.0877) radius 0.5023
  circle A734 centre (-10.7365, -34.7386) radius 0.5023
  circle A735 centre (-10.7365, -38.3895) radius 0.5023
  circle A736 centre (-10.7365, -42.0405) radius 0.5023
  circle A737 centre (-10.7365, -45.6914) radius 0.5023
  circle A738 centre (-10.7365, -49.3423) radius 0.5023
  circle A739 centre (-10.7365, -52.9933) radius 0.5023
  circle A740 centre (-10.7365, -56.6442) radius 0.5023
  circle A741 centre (-10.7365, -60.2951) radius 0.5023
  circle A742 centre (-10.7365, -63.9461) radius 0.5023
  circle A743 centre (-10.7365, -67.597) radius 0.5023
  circle A744 centre (-10.7365, -71.248) radius 0.5023
  circle A745 centre (-10.7365, -74.8989) radius 0.5023
  circle A746 centre (-10.7365, -78.5498) radius 0.5023
  circle A747 centre (-10.7365, -82.2008) radius 0.5023
  circle A748 centre (-10.7365, -85.8517) radius 0.5023
  circle A749 centre (-10.7365, -89.5026) radius 0.5023
  circle A750 centre (-10.7365, -93.1536) radius 0.5023
  circle A751 centre (-10.7365, -96.8045) radius 0.5023
  circle A752 centre (-10.7365, -100.4554) radius 0.5023
  circle A753 centre (-10.7365, -104.1064) radius 0.5023
  circle A754 centre (-10.7365, -107.7573) radius 0.5023
  circle A755 centre (-10.7365, -111.4082) radius 0.5023
  circle A756 centre (-10.7365, -115.0592) radius 0.5023
  circle A757 centre (-10.7365, -118.7101) radius 0.5023
  circle A758 centre (-10.7365, -122.361) radius 0.5023
  circle A759 centre (-10.7365, -126.012) radius 0.5023
  circle A760 centre (-10.7365, -129.6629) radius 0.5023
  circle A761 centre (-10.7365, -133.3138) radius 0.5023
  circle A762 centre (-10.7365, -136.9648) radius 0.5023
  circle A763 centre (-10.7365, -140.6157) radius 0.5023
  circle A764 centre (-10.7365, -144.2667) radius 0.5023
  circle A765 centre (-10.7365, -147.9176) radius 0.5023
  circle A766 centre (-10.7365, -151.5685) radius 0.5023
  circle A767 centre (-10.7365, -155.2195) radius 0.5023
  circle A768 centre (-10.7365, -158.8704) radius 0.5023
  circle A769 centre (-10.7365, -162.5213) radius 0.5023
  circle A770 centre (-10.7365, -166.1723) radius 0.5023
  circle A771 centre (-10.7365, -169.8232) radius 0.5023
  circle A772 centre (-10.7365, -173.4741) radius 0.5023
  circle A773 centre (-10.7365, -177.1251) radius 0.5023
  circle A774 centre (-10.7365, -180.776) radius 0.5023
  circle A775 centre (-10.7365, -184.4269) radius 0.5023
  circle A776 centre (-10.7365, -188.0779) radius 0.5023
  circle A777 centre (-10.7365, -191.7288) radius 0.5023
  circle A778 centre (-10.7365, -195.3797) radius 0.5023
  circle A779 centre (-10.7365, -199.0307) radius 0.5023
  circle A780 centre (-10.7365, -202.6816) radius 0.5023
  circle A781 centre (-10.7365, -206.3325) radius 0.5023
  circle A782 centre (-10.7365, -209.9835) radius 0.5023
  circle A783 centre (-10.7365, -213.6344) radius 0.5023
  circle A784 centre (-10.7365, -217.2853) radius 0.5023
  circle A785 centre (-10.7365, -220.9363) radius 0.5023
  circle A786 centre (-10.7365, -224.5872) radius 0.5023
  circle A787 centre (-12.5458, -7.3404) radius 0.5023
  circle A788 centre (-12.5458, -10.9913) radius 0.5023
  circle A789 centre (-12.5458, -14.6422) radius 0.5023
  circle A790 centre (-12.5458, -18.2932) radius 0.5023
  circle A791 centre (-12.5458, -21.9441) radius 0.5023
  circle A792 centre (-12.5458, -25.595) radius 0.5023
  circle A793 centre (-12.5458, -29.246) radius 0.5023
  circle A794 centre (-12.5458, -32.8969) radius 0.5023
  circle A795 centre (-12.5458, -36.5478) radius 0.5023
  circle A796 centre (-12.5458, -40.1988) radius 0.5023
  circle A797 centre (-12.5458, -43.8497) radius 0.5023
  circle A798 centre (-12.5458, -47.5006) radius 0.5023
  circle A799 centre (-12.5458, -51.1516) radius 0.5023
  circle A800 centre (-12.5458, -54.8025) radius 0.5023
  circle A801 centre (-12.5458, -58.4534) radius 0.5023
  circle A802 centre (-12.5458, -62.1044) radius 0.5023
  circle A803 centre (-12.5458, -65.7553) radius 0.5023
  circle A804 centre (-12.5458, -69.4062) radius 0.5023
  circle A805 centre (-12.5458, -73.0572) radius 0.5023
  circle A806 centre (-12.5458, -76.7081) radius 0.5023
  circle A807 centre (-12.5458, -80.3591) radius 0.5023
  circle A808 centre (-12.5458, -84.01) radius 0.5023
  circle A809 centre (-12.5458, -87.6609) radius 0.5023
  circle A810 centre (-12.5458, -91.3119) radius 0.5023
  circle A811 centre (-12.5458, -94.9628) radius 0.5023
  circle A812 centre (-12.5458, -98.6137) radius 0.5023
  circle A813 centre (-12.5458, -102.2647) radius 0.5023
  circle A814 centre (-12.5458, -105.9156) radius 0.5023
  circle A815 centre (-12.5458, -109.5665) radius 0.5023
  circle A816 centre (-12.5458, -113.2175) radius 0.5023
  circle A817 centre (-12.5458, -116.8684) radius 0.5023
  circle A818 centre (-12.5458, -120.5193) radius 0.5023
  circle A819 centre (-12.5458, -124.1703) radius 0.5023
  circle A820 centre (-12.5458, -127.8212) radius 0.5023
  circle A821 centre (-12.5458, -131.4721) radius 0.5023
  circle A822 centre (-12.5458, -135.1231) radius 0.5023
  circle A823 centre (-12.5458, -138.774) radius 0.5023
  circle A824 centre (-12.5458, -142.4249) radius 0.5023
  circle A825 centre (-12.5458, -146.0759) radius 0.5023
  circle A826 centre (-12.5458, -149.7268) radius 0.5023
  circle A827 centre (-12.5458, -153.3778) radius 0.5023
  circle A828 centre (-12.5458, -157.0287) radius 0.5023
  circle A829 centre (-12.5458, -160.6796) radius 0.5023
  circle A830 centre (-12.5458, -164.3306) radius 0.5023
  circle A831 centre (-12.5458, -167.9815) radius 0.5023
  circle A832 centre (-12.5458, -171.6324) radius 0.5023
  circle A833 centre (-12.5458, -175.2834) radius 0.5023
  circle A834 centre (-12.5458, -178.9343) radius 0.5023
  circle A835 centre (-12.5458, -182.5852) radius 0.5023
  circle A836 centre (-12.5458, -186.2362) radius 0.5023
  circle A837 centre (-12.5458, -189.8871) radius 0.5023
  circle A838 centre (-12.5458, -193.538) radius 0.5023
  circle A839 centre (-12.5458, -197.189) radius 0.5023
  circle A840 centre (-12.5458, -200.8399) radius 0.5023
  circle A841 centre (-12.5458, -204.4908) radius 0.5023
  circle A842 centre (-12.5458, -208.1418) radius 0.5023
  circle A843 centre (-12.5458, -211.7927) radius 0.5023
  circle A844 centre (-12.5458, -215.4436) radius 0.5023
  circle A845 centre (-12.5458, -219.0946) radius 0.5023
  circle A846 centre (-12.5458, -222.7455) radius 0.5023
  circle A847 centre (-15.0186, -5.5311) radius 0.5023
  circle A848 centre (-15.0186, -9.1821) radius 0.5023
  circle A849 centre (-15.0186, -12.833) radius 0.5023
  circle A850 centre (-15.0186, -16.4839) radius 0.5023
  circle A851 centre (-15.0186, -20.1349) radius 0.5023
  circle A852 centre (-15.0186, -23.7858) radius 0.5023
  circle A853 centre (-15.0186, -27.4367) radius 0.5023
  circle A854 centre (-15.0186, -31.0877) radius 0.5023
  circle A855 centre (-15.0186, -34.7386) radius 0.5023
  circle A856 centre (-15.0186, -38.3895) radius 0.5023
  circle A857 centre (-15.0186, -42.0405) radius 0.5023
  circle A858 centre (-15.0186, -45.6914) radius 0.5023
  circle A859 centre (-15.0186, -49.3423) radius 0.5023
  circle A860 centre (-15.0186, -52.9933) radius 0.5023
  circle A861 centre (-15.0186, -56.6442) radius 0.5023
  circle A862 centre (-15.0186, -60.2951) radius 0.5023
  circle A863 centre (-15.0186, -63.9461) radius 0.5023
  circle A864 centre (-15.0186, -67.597) radius 0.5023
  circle A865 centre (-15.0186, -71.248) radius 0.5023
  circle A866 centre (-15.0186, -74.8989) radius 0.5023
  circle A867 centre (-15.0186, -78.5498) radius 0.5023
  circle A868 centre (-15.0186, -82.2008) radius 0.5023
  circle A869 centre (-15.0186, -85.8517) radius 0.5023
  circle A870 centre (-15.0186, -89.5026) radius 0.5023
  circle A871 centre (-15.0186, -93.1536) radius 0.5023
  circle A872 centre (-15.0186, -96.8045) radius 0.5023
  circle A873 centre (-15.0186, -100.4554) radius 0.5023
  circle A874 centre (-15.0186, -104.1064) radius 0.5023
  circle A875 centre (-15.0186, -107.7573) radius 0.5023
  circle A876 centre (-15.0186, -111.4082) radius 0.5023
  circle A877 centre (-15.0186, -115.0592) radius 0.5023
  circle A878 centre (-15.0186, -118.7101) radius 0.5023
  circle A879 centre (-15.0186, -122.361) radius 0.5023
  circle A880 centre (-15.0186, -126.012) radius 0.5023
  circle A881 centre (-15.0186, -129.6629) radius 0.5023
  circle A882 centre (-15.0186, -133.3138) radius 0.5023
  circle A883 centre (-15.0186, -136.9648) radius 0.5023
  circle A884 centre (-15.0186, -140.6157) radius 0.5023
  circle A885 centre (-15.0186, -144.2667) radius 0.5023
  circle A886 centre (-15.0186, -147.9176) radius 0.5023
  circle A887 centre (-15.0186, -151.5685) radius 0.5023
  circle A888 centre (-15.0186, -155.2195) radius 0.5023
  circle A889 centre (-15.0186, -158.8704) radius 0.5023
  circle A890 centre (-15.0186, -162.5213) radius 0.5023
  circle A891 centre (-15.0186, -166.1723) radius 0.5023
  circle A892 centre (-15.0186, -169.8232) radius 0.5023
  circle A893 centre (-15.0186, -173.4741) radius 0.5023
  circle A894 centre (-15.0186, -177.1251) radius 0.5023
  circle A895 centre (-15.0186, -180.776) radius 0.5023
  circle A896 centre (-15.0186, -184.4269) radius 0.5023
  circle A897 centre (-15.0186, -188.0779) radius 0.5023
  circle A898 centre (-15.0186, -191.7288) radius 0.5023
  circle A899 centre (-15.0186, -195.3797) radius 0.5023
  circle A900 centre (-15.0186, -199.0307) radius 0.5023
  circle A901 centre (-15.0186, -202.6816) radius 0.5023